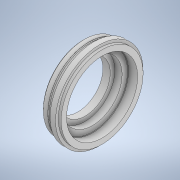
# Autodesk Inventor part: Крышка тих_выход
Saved by Autodesk Inventor 2021 (Build 250183000, 183)
## iProperties
Created: 2023-03-17
Part Number: Крышка тих_выход
Material: Типовые
Document SubType Name: Modeling
Designer: gdevc
Density: 1 g/cm^3
Appearance: По умолчанию
Mass: 48.6347 g
Surface Area: 182.136 cm^2
Volume: 48.6347 cm^3
Author: gdevc
Autodesk Inventor part; units mm, degrees
ref_plane "YZ Plane" through (0, 0, 0) normal (1, 0, 0) x (0, 1, 0)
ref_plane "XZ Plane" through (0, 0, 0) normal (0, 1, 0) x (-1, 0, 0)
ref_plane "XY Plane" through (0, 0, 0) normal (0, 0, 1) x (1, 0, 0)
sketch "Эскиз1" plane through (0, 0, 0) normal (0, 0, 1) x (1, 0, 0)
  line L0 (0, 27.5) -> (0, 45)
  line L1 (0, 45) -> (6, 45)
  line L2 (6, 45) -> (6.5, 44.5)
  line L3 (6.5, 44.5) -> (11.5, 44.5)
  line L4 (11.5, 44.5) -> (11.5, 48)
  line L5 (11.5, 48) -> (17.5, 48)
  line L6 (17.5, 48) -> (17.5, 45)
  line L7 (17.5, 39) -> (10, 39)
  line L8 (10, 39) -> (10, 32.5)
  line L9 (10, 32.5) -> (2, 32.5)
  line L10 (2, 32.5) -> (2, 27.5)
  line L11 (2, 27.5) -> (0, 27.5)
  line L12 (0, 0) -> (122.1011, 0) construction
  line L13 (17.5, 45) -> (20.55, 45)
  line L14 (20.55, 45) -> (20.55, 39)
  line L15 (20.55, 39) -> (17.5, 39)
  dimension "d0" = 90
  dimension "d1" = 65
  dimension "d2" = 5
  dimension "d4" = 5
  dimension "d5" = 6
  dimension "d7" = 45
  dimension "d8" = 0.5
  dimension "d9" = 9
  dimension "d10" = 6
  dimension "d12" = 2
  dimension "d19" = 96
  dimension "d20" = 10
  dimension "d24" = 3.05
  constraints: 32 end point, 9 perpendicular, 2 horizontal, 2 point on line, 2 vertical, 1 parallel, 1 vertical alignment
  measures "d0" diameter of L1 L12
  measures "d1" diameter of L9 L12
  measures "d2" distance between parallel lines of L11 L9
  measures "d4" distance of L2.end L3.end
  measures "d5" distance of L0.end L1.end
  measures "d7" angle of L3 L2
  measures "d8" distance between parallel lines of L1 L3
  measures "d9" distance between parallel lines of L7 L5
  measures "d10" distance of L4.end L5.end
  measures "d12" distance of L10.end L0.start
  measures "d19" diameter of L5 L12
  measures "d20" distance between parallel lines of L0 L8
  measures "d24" distance of L6.end L13.end
revolve "Вращение1" add sketch "Эскиз1" angle 360 about axis through (0, 0, 0) along (1, 0, 0)
fillet "Сопряжение1" radius 1.6 2 edges at (6.5, -44.5, 0) (11.5, -44.5, 0)
chamfer "Фаска1" distance 1 angle 45 1 edges at (0, -45, 0)
fillet "Сопряжение2" radius 0.5 1 edges at (10, -39, 0)
sketch "Эскиз2" plane through (0, 0, 0) normal (-1, 0, 0) x (0, 0, 1)
  circle A0 centre (0, 0) radius 27.5 projected
  circle A1 centre (0, 0) radius 33.5
  dimension "d21" = 6
  constraints: 1 centre point, 1 coincident
  measures "d21" radial gap between concentric circles of A1 A0
extrude "Выдавливание1" add sketch "Эскиз2" along normal blind 6
